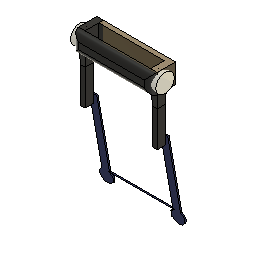
walking assist square exterior (Autodesk Fusion 360 design; units mm, degrees)
Autodesk Fusion 360 part; units mm, degrees
note: some values were not read from the file. Chosen so that the rebuilt part matches the saved one: which bodies a step acts on; which face or edge a step refers to. Set by a fixed rule: which sketch regions a step uses.
sketch "Sketch1" plane through (0, 0, 0) normal (1, 0, 0) x (0, 1, 0)
  line L0 (-85, 75) -> (75, 75)
  line L1 (75, 75) -> (75, -75)
  line L2 (75, -75) -> (-85, -75)
  line L3 (-85, -75) -> (-85, 75)
  constraint perpendicular L0 L1
  constraint parallel L0 L2
  constraint parallel L1 L3
  constraint horizontal L0
extrude "Extrude1" add sketch "Sketch1" along normal blind 800 makes body 1
extrude "Extrude2" cut 1 faces at (800, -31.6667, -25) along direction (-1, 0, 0) blind 200 on bodies 1 bodies 1
fillet "Fillet1" radius 50 1 faces at (200, -85, -25) on bodies 1
ref_plane "WorkPlane1" through (-25, -5, 0) normal (-1, 0, 0) x (0, -1, 0)
sketch "Sketch2" plane through (-25, 0, 0) normal (-1, 0, 0) x (0, -1, 0)
  circle A0 centre (0, 0) radius 70
  dimension "d8" = 140
  constraint coincident A0.centre origin
  measures "d8" diameter of A0
extrude "Extrude3" add sketch "Sketch2" against normal blind 50 separate body makes body 2
ref_plane "WorkPlane2" through (625, -5, 0) normal (1, 0, 0) x (0, 0, -1)
sketch "Sketch3" plane through (625, 0, 0) normal (1, 0, 0) x (0, 1, 0)
  circle A0 centre (0, 0) radius 70
  dimension "d12" = 140
  constraint coincident A0.centre origin
  measures "d12" diameter of A0
extrude "Extrude4" add sketch "Sketch3" against normal blind 50 separate body makes body 3
sketch "Sketch4" plane through (0, 0, 75) normal (0, 0, 1) x (-1, 0, 0)
  line L0 (0, 35) -> (-600, 35)
  line L1 (-600, 35) -> (-600, -75)
  line L2 (-600, -75) -> (0, -75)
  line L3 (0, -75) -> (0, 35)
  line L4 (-550, 35) -> (-49.7203, 35)
  line L5 (-49.7203, 35) -> (-49.7203, -75)
  line L6 (-49.7203, -75) -> (-550, -75)
  line L7 (-550, -75) -> (-550, 35)
  constraint horizontal L4
  constraint vertical L5
  constraint horizontal L6
  constraint vertical L7
  constraint coincident L2 L5.end
  constraint coincident L0 L4.start
extrude "Extrude5" cut sketch "Sketch4" along normal mid plane 580 contours L0 L2 L4 L5 L6 L7 bodies 1
extrude "Extrude6" add 1 faces at (33.1469, 38.3333, -75) along direction (0, 0, -1) blind 100 draft -5 on bodies 1 bodies 1
extrude "Extrude7" add 1 faces at (566.6667, 38.3333, -75) along direction (0, 0, -1) blind 100 draft -5 on bodies 1 bodies 1
extrude "Extrude8" add 1 faces at (30.2306, 35.417, -175) along direction (0, 0, -1) blind 200 on bodies 1 bodies 1
extrude "Extrude9" add 1 faces at (30.2306, 35.417, -375) along direction (0, 0, -1) blind 50 on bodies 1 bodies 1
extrude "Extrude10" add 1 faces at (569.583, 35.417, -175) along direction (0, 0, -1) blind 270 on bodies 1 bodies 1
extrude "Extrude11" add 1 faces at (30.2306, 35.417, -425) along direction (0, 0, -1) blind 5 on bodies 1 bodies 1
extrude "Extrude12" add 1 faces at (30.2306, 35.417, -430) along direction (0, 0, -1) blind 5 on bodies 1 bodies 1
extrude "Extrude13" add 1 faces at (30.2306, 35.417, -435) along direction (0, 0, -1) blind 10 on bodies 1 bodies 1
extrude "Extrude14" add 1 faces at (566.6667, 75, 25) along direction (0, 1, 0) blind 50 on bodies 1 bodies 1
extrude "Extrude15" add 1 faces at (16.5734, 75, 25) along direction (0, 1, 0) blind 50 on bodies 1 bodies 1
extrude "Extrude16" add 1 faces at (566.6667, 91.6667, -75) along direction (0, 0, -1) blind 1000 on bodies 1 bodies 1
extrude "Extrude17" add 1 faces at (16.5734, 91.6667, -75) along direction (0, 0, -1) blind 1000 on bodies 1 bodies 1
sketch "Sketch5" plane through (550, 0, 0) normal (-1, 0, 0) x (0, -1, 0)
  line L0 (-75, -75) -> (35, -75)
  line L1 (35, -75) -> (35, 75)
  line L2 (35, 75) -> (-125, 75)
  line L3 (-125, 75) -> (-125, -1075)
  line L4 (-125, -1075) -> (-75, -1075)
  line L5 (-75, -1075) -> (-75, -75)
  line L6 (-75, -1075) -> (-125, -1075)
  line L7 (-125, -1075) -> (-125, -1025)
  line L8 (-125, -1025) -> (-75, -1025)
  line L9 (-75, -1025) -> (-75, -1075)
  constraint horizontal L6
  constraint vertical L7
  constraint horizontal L8
  constraint vertical L9
  constraint coincident L3 L7.end
  constraint coincident L4.end L5.start
extrude "Extrude18" add sketch "Sketch5" along normal blind 550 separate body contours L3 L4 L5 L6 L7 L8 L9 makes body 4
sketch "Sketch6" plane through (0, 125, 0) normal (0, 1, 0) x (-1, 0, 0)
  line L0 (-550, -1025) -> (-550, -1075)
  line L1 (-550, -1075) -> (0, -1075)
  line L2 (0, -1075) -> (0, -1025)
  line L3 (0, -1025) -> (-550, -1025)
  circle A0 centre (-575, -1050) radius 50
  dimension "d43" = 100
  measures "d43" diameter of A0
extrude "Extrude19" add sketch "Sketch6" against normal blind 50 separate body contours L0 L1 L3 A0 picked at (-574.9534, -1048.7545) makes body 5
sketch "Sketch7" plane through (0, 125, 0) normal (0, 1, 0) x (-1, 0, 0)
  line L0 (-550, -1025) -> (-550, -1075)
  line L1 (-550, -1075) -> (0, -1075)
  line L2 (0, -1075) -> (0, -1025)
  line L3 (0, -1025) -> (-550, -1025)
  circle A0 centre (-25, -1050) radius 50
  dimension "d46" = 100
  measures "d46" diameter of A0
extrude "Extrude20" add sketch "Sketch7" against normal blind 50 separate body contours L1 L2 L3 A0 | L1 L2 L3 A0 makes body 6
sketch "Sketch8" plane through (0, 125, 0) normal (0, 1, 0) x (-1, 0, 0)
  line L0 (-550, -1075) -> (-550, 75)
  line L1 (-550, 75) -> (-600, 75)
  line L2 (-600, 75) -> (-600, -1075)
  line L3 (-600, -1075) -> (-550, -1075)
  line L4 (-700, -500) -> (100, -500)
  line L5 (100, -500) -> (100, -1000)
  line L6 (100, -1000) -> (-700, -1000)
  line L7 (-700, -1000) -> (-700, -500)
  constraint horizontal L4
  constraint vertical L5
  constraint horizontal L6
  constraint vertical L7
extrude "Extrude21" cut sketch "Sketch8" against normal blind 200 contours L0 L4 L5 L6 | L2 L4 L6 L7 bodies 1 makes body 7 at (0, 91.6667, -1025)
sketch "Sketch9" plane through (0, 0, 0) normal (0, 1, 0) x (1, 0, 0)
  line L0 (-102.96, 450.4498, -26.2511) -> (852.6372, 450.4498, -26.2511)
  line L1 (852.6372, 450.4498, -26.2511) -> (852.6372, 997.4246, -26.2511)
  line L2 (852.6372, 997.4246, -26.2511) -> (-102.96, 997.4246, -26.2511)
  line L3 (-102.96, 997.4246, -26.2511) -> (-102.96, 450.4498, -26.2511)
sketch "Sketch9 (curves -26.2511 mm off its plane)" plane through (0, -26.2511, 0) normal (0, 1, 0) x (1, 0, 0)
  line L0 (-102.96, 450.4498) -> (852.6372, 450.4498)
  line L1 (852.6372, 450.4498) -> (852.6372, 997.4246)
  line L2 (852.6372, 997.4246) -> (-102.96, 997.4246)
  line L3 (-102.96, 997.4246) -> (-102.96, 450.4498)
extrude "Extrude22" cut sketch "Sketch9 (curves -26.2511 mm off its plane)" along normal blind 500 bodies 1 makes body 8 at (550, 91.6667, -1023.2831)
extrude "Extrude23" cut 1 faces at (566.6667, 91.6667, -450.4498) along direction (0, 0, 1) blind 550 on bodies 1 bodies 1
extrude "Extrude24" cut 1 faces at (16.5734, 91.6667, -450.4498) along direction (0, 0, 1) blind 600 on bodies 1 bodies 1
extrude "Extrude25" cut 1 faces at (366.6667, 125, -1041.6667) along direction (0, -1, 0) blind 150 on bodies 4 bodies 4 6 7
extrude "Extrude26" add 1 faces at (45.5342, 108.3333, -1025) along direction (0, 0, -1) blind 50 on bodies 6 bodies 4 6 7
extrude "Extrude27" add 1 faces at (550, 108.3333, -1041.6667) along direction (-1, 0, 0) blind 10 on bodies 5 bodies 5 8
extrude "Extrude28" add 1 faces at (534.4658, 108.3333, -1025) along direction (0, 0, -1) blind 50 on bodies 5 bodies 5
extrude "Extrude29" cut 1 faces at (566.6667, 108.3333, -997.4246) along direction (0, 0, -1) blind 5 on bodies 5 bodies 5
extrude "Extrude30" cut 1 faces at (16.5734, 108.3333, -1000) along direction (0, 0, -1) blind 5 on bodies 4 bodies 4
extrude "Extrude31" add 1 faces at (68.3013, 108.3333, -1058.3333) along direction (1, 0, 0) blind 10 on bodies 4 bodies 4
extrude "Extrude32" add 1 faces at (531.6987, 108.3333, -1058.3333) along direction (-1, 0, 0) blind 10 on bodies 5 bodies 5
extrude "Extrude33" add 1 faces at (566.6667, 108.3333, -1002.4246) along direction (0, 0, 1) blind 10 on bodies 5 bodies 5
extrude "Extrude34" add 1 faces at (16.5734, 108.3333, -1005) along direction (0, 0, 1) blind 10 on bodies 4 bodies 4
extrude "Extrude35" add 1 faces at (550, 91.6667, -997.1827) along direction (-1, 0, 0) blind 550 on bodies 5 bodies 4 5
extrude "Extrude36" add 1 faces at (200, 91.6667, -992.4246) along direction (0, 0, 1) blind 1100 on bodies 4 bodies 1 2 3 4
sketch "Sketch10" plane through (0, 0, 0) normal (0, 1, 0) x (1, 0, 0)
  line L0 (57.7541, 100.2204) -> (541.9927, 100.2204)
  line L1 (541.9927, 100.2204) -> (541.9927, 1006.3918)
  line L2 (541.9927, 1006.3918) -> (57.7541, 1006.3918)
  line L3 (57.7541, 1006.3918) -> (57.7541, 100.2204)
  constraint horizontal L0
  constraint vertical L1
  constraint horizontal L2
  constraint vertical L3
extrude "Extrude37" cut sketch "Sketch10" along normal blind 300 bodies 1
extrude "Extrude38" cut 1 faces at (216.4802, 75, 25) along direction (0, -1, 0) blind 40 on bodies 1 bodies 1
extrude "Extrude39" cut 1 faces at (216.4802, 75, 25) along direction (0, 1, 0) blind 30 on bodies 1 bodies 1
extrude "Extrude40" cut 1 faces at (400, 118.3333, 107.5754) along direction (0, 0, -1) blind 550 on bodies 1 bodies 1 makes body 9 at (563.9976, 105, -630.516)
extrude "Extrude41" cut 1 faces at (563.9976, 105, -630.516) along direction (0, 1, 0) blind 10 on bodies 9 bodies 9
move_body "Move1" bodies 9 to x (1, 0, 0) y (0, 0.984808, 0.173648) z (0, -0.173648, 0.984808) at (3.7084, -148.0483, 30.5857)
sketch "Sketch11" plane through (550, 0, 0) normal (-1, 0, 0) x (0, -1, 0)
  line L0 (-35, -75) -> (35, -75)
  line L1 (35, -75) -> (35, 75)
  line L2 (35, 75) -> (-105, 75)
  line L3 (-105, 75) -> (-105, -75)
  line L4 (-105, -75) -> (-35, -75)
  line L5 (-105, 75) -> (-70, 75)
  line L6 (-70, 75) -> (-70, -75)
  line L7 (-70, -75) -> (-105, -75)
  line L8 (-105, -75) -> (-105, 75)
  constraint horizontal L5
  constraint vertical L6
  constraint horizontal L7
  constraint vertical L8
  constraint midpoint L4 L6.end
  constraint coincident L2.end L3.start
extrude "Extrude42" add sketch "Sketch11" along normal blind 500 contours L2 L3 L4 L5 L6 L7 L8 bodies 1
